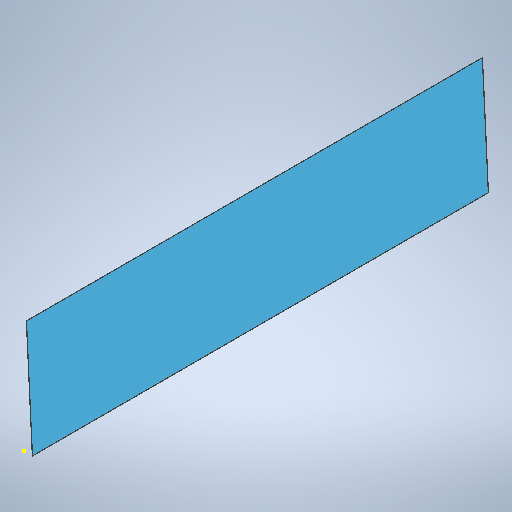
# Autodesk Inventor part: GBK-Dummy wall1
Saved by Autodesk Inventor 2026.2 (Build 302298000, 298)
## iProperties
Created: 2026-05-13
Part Number: GBK-Dummy wall1
Material: Generic
Document SubType Name: Modeling
Designer: admin
Density: 1 g/cm^3
Appearance: Default
Author: admin
Autodesk Inventor part; units mm, degrees
ref_plane "YZ Plane" through (0, 0, 0) normal (1, 0, 0) x (0, 1, 0)
ref_plane "XZ Plane" through (0, 0, 0) normal (0, 1, 0) x (-1, 0, 0)
ref_plane "XY Plane" through (0, 0, 0) normal (0, 0, 1) x (1, 0, 0)
sketch "Sketch1" plane through (0, 0, 0) normal (0, 0, 1) x (1, 0, 0)
  line L0 (355.835, 0) -> (345.835, 0)
  line L1 (345.835, 0) -> (110.0274, 4499.4774)
  line L2 (110.0274, 4499.4774) -> (120, 4500)
  line L3 (120, 4500) -> (355.835, 0)
  line L4 (0, 4500) -> (0, 0)
  dimension "d0" = 10
  dimension "d1" = 87
  dimension "d2" = 4500
  dimension "d5" = 120
  constraints: 10 end point, 2 perpendicular, 1 horizontal, 1 horizontal alignment, 1 point on line, 1 vertical
  measures "d0" distance of L0.start L0.end
  measures "d1" angle of L0 L1
  measures "d2" distance from line of L0 L2.end
  measures "d5" distance of L2.end L4.start
extrude "Extrusion1" add sketch "Sketch1" against normal blind 18000
sketch "Sketch2" plane through (0, 0, 0) normal (1, 0, 0) x (0, 1, 0)
  point P0 (0, 0)
body "Solid1"
